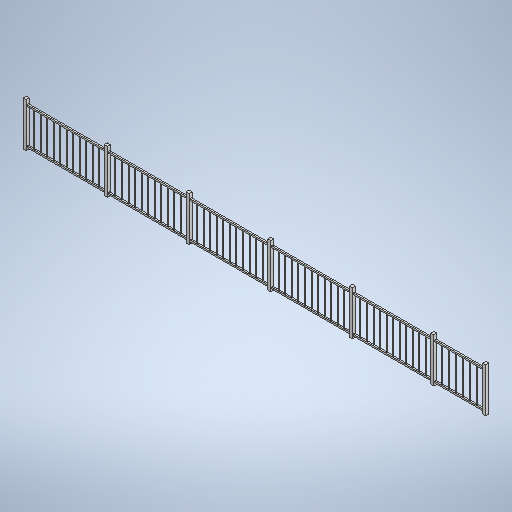
# Autodesk Inventor part: Railing Side B
Saved by Autodesk Inventor 2025 (Build 290162000, 162)
## iProperties
Created: 2024-07-15
Part Number: Railing Side B
Material: Generic
Document SubType Name: Modeling
Designer: track
Density: 1 g/cm^3
Appearance: Default
Author: track
Autodesk Inventor part; units mm, degrees
ref_plane "YZ Plane" through (0, 0, 0) normal (1, 0, 0) x (0, 1, 0)
ref_plane "XZ Plane" through (0, 0, 0) normal (0, 1, 0) x (-1, 0, 0)
ref_plane "XY Plane" through (0, 0, 0) normal (0, 0, 1) x (1, 0, 0)
sketch "Sketch1" plane through (0, 0, 0) normal (0, 1, 0) x (-1, 0, 0)
  line L0 (-38.1, -38.1) -> (38.1, -38.1)
  line L1 (38.1, -38.1) -> (38.1, 38.1)
  line L2 (38.1, 38.1) -> (-38.1, 38.1)
  line L3 (-38.1, 38.1) -> (-38.1, -38.1)
  line L4 (-38.1, -38.1) -> (38.1, 38.1) construction
  line L5 (38.1, -38.1) -> (-38.1, 38.1) construction
  point P0 (0, 0)
  dimension "d0" = 76.2
  dimension "d1" = 76.2
  constraints: 12 end point, 2 midpoint, 2 parallel, 1 horizontal, 1 perpendicular
  measures "d0" distance of L1.end L2.end
  measures "d1" distance of L0.end L1.end
extrude "Extrusion1" add sketch "Sketch1" along normal blind 1117.6
sketch "Sketch2" plane through (38.1, 0, 38.1) normal (1, 0, 0) x (0, 0, -1)
  line L0 (19.05, 95.25) -> (57.15, 95.25)
  line L1 (57.15, 95.25) -> (57.15, 57.15)
  line L2 (57.15, 57.15) -> (19.05, 57.15)
  line L3 (19.05, 57.15) -> (19.05, 95.25)
  line L4 (19.05, 95.25) -> (57.15, 57.15) construction
  line L5 (57.15, 95.25) -> (19.05, 57.15) construction
  line L6 (19.05, 996.95) -> (57.15, 996.95)
  line L7 (57.15, 996.95) -> (57.15, 958.85)
  line L8 (57.15, 958.85) -> (19.05, 958.85)
  line L9 (19.05, 958.85) -> (19.05, 996.95)
  line L10 (19.05, 996.95) -> (57.15, 958.85) construction
  line L11 (57.15, 996.95) -> (19.05, 958.85) construction
  line L12 (76.2, 329.1929) -> (76.2, 1461.8329)
  line L13 (76.2, 282.1305) -> (76.2, 1152.2607)
  line L14 (76.2, 0) -> (76.2, 1117.6) projected
  line L15 (0, 0) -> (76.2, 0) projected
  point P0 (38.1, 0)
  point P1 (-393.2293, 273.1932)
  point P2 (483.6892, 252.9929)
  point P3 (38.1, 76.2)
  point P4 (38.1, 977.9)
  dimension "d4" = 38.1
  dimension "d5" = 38.1
  dimension "d6" = 38.1
  dimension "d7" = 863.6
  dimension "d8" = 38.1
  dimension "d9" = 38.1
  dimension "d10" = 38.1
  dimension "d12" = 76.2
  constraints: 28 end point, 4 midpoint, 4 parallel, 2 horizontal, 2 perpendicular, 1 collinear, 1 point on line, 1 vertical
  measures "d4" distance of L0.end L1.end
  measures "d5" distance of L0.start L0.end
  measures "d6" distance from line of L12 point (38.1, 76.2)
  measures "d7" distance between parallel lines of L8 L0
  measures "d8" distance of L6.end L7.end
  measures "d9" distance of L6.start L6.end
  measures "d10" distance from line of L13 point (38.1, 977.9)
  measures "d12" distance from line of L15 point (38.1, 76.2)
extrude "Extrusion2" add sketch "Sketch2" along normal blind 1971.675
sketch "Sketch3" plane through (0, 0, 0) normal (0, 1, 0) x (-1, 0, 0)
  line L0 (0, 0) -> (-2047.875, 0)
  line L1 (-38.1, -19.05) -> (-2009.775, -19.05) projected
  line L2 (-2009.775, 38.1) -> (-2085.975, 38.1)
  line L3 (-2085.975, 38.1) -> (-2085.975, -38.1)
  line L4 (-2085.975, -38.1) -> (-2009.775, -38.1)
  line L5 (-2009.775, -38.1) -> (-2009.775, 38.1)
  line L6 (-2009.775, 38.1) -> (-2085.975, -38.1) construction
  line L7 (-2085.975, 38.1) -> (-2009.775, -38.1) construction
  line L8 (-2009.775, -19.05) -> (-2009.775, 19.05) projected
  dimension "d15" = 76.2
  dimension "d16" = 76.2
  constraints: 14 end point, 3 parallel, 2 midpoint, 1 collinear, 1 horizontal, 1 perpendicular
  measures "d15" distance of L3.end L4.end
  measures "d16" distance of L2.end L3.end
extrude "Extrusion3" add sketch "Sketch3" along normal blind 1117.6
sketch "Sketch4" plane through (2085.975, 0, 38.1) normal (1, 0, 0) x (0, 0, -1)
  line L0 (57.15, 996.95) -> (57.15, 958.85) projected
  line L1 (57.15, 958.85) -> (57.15, 996.95) projected
  line L2 (19.05, 996.95) -> (57.15, 996.95) projected
  line L3 (57.15, 996.95) -> (19.05, 996.95) projected
  line L4 (19.05, 958.85) -> (19.05, 996.95) projected
  line L5 (19.05, 996.95) -> (19.05, 958.85) projected
  line L6 (57.15, 958.85) -> (19.05, 958.85) projected
  line L7 (19.05, 958.85) -> (57.15, 958.85) projected
  line L8 (57.15, 57.15) -> (19.05, 57.15) projected
  line L9 (19.05, 57.15) -> (57.15, 57.15) projected
  line L10 (19.05, 57.15) -> (19.05, 95.25) projected
  line L11 (19.05, 95.25) -> (19.05, 57.15) projected
  line L12 (19.05, 95.25) -> (57.15, 95.25) projected
  line L13 (57.15, 95.25) -> (19.05, 95.25) projected
  line L14 (57.15, 95.25) -> (57.15, 57.15) projected
  line L15 (57.15, 57.15) -> (57.15, 95.25) projected
  line L16 (19.05, 95.25) -> (57.15, 95.25)
  line L17 (57.15, 95.25) -> (57.15, 57.15)
  line L18 (57.15, 57.15) -> (19.05, 57.15)
  line L19 (19.05, 57.15) -> (19.05, 95.25)
  line L20 (19.05, 996.95) -> (57.15, 996.95)
  line L21 (57.15, 996.95) -> (57.15, 958.85)
  line L22 (57.15, 958.85) -> (19.05, 958.85)
  line L23 (19.05, 958.85) -> (19.05, 996.95)
  point P0 (38.1, 0)
  point P1 (19.05, 958.85)
  point P2 (57.15, 958.85)
  point P3 (57.15, 996.95)
  point P4 (19.05, 996.95)
  point P5 (57.15, 57.15)
  point P6 (57.15, 95.25)
  point P7 (19.05, 95.25)
  point P8 (19.05, 57.15)
  constraints: 16 end point, 4 parallel, 2 horizontal, 2 perpendicular
extrude "Extrusion4" add sketch "Sketch4" along normal blind 1985.9625
sketch "Sketch5" plane through (0, 0, 0) normal (0, 1, 0) x (-1, 0, 0)
  line L0 (-4071.9375, -19.05) -> (-4071.9375, 19.05) projected
  line L1 (-4071.9375, 0) -> (-4110.0375, 0)
  line L2 (-4148.1375, -38.1) -> (-4071.9375, -38.1)
  line L3 (-4071.9375, -38.1) -> (-4071.9375, 38.1)
  line L4 (-4071.9375, 38.1) -> (-4148.1375, 38.1)
  line L5 (-4148.1375, 38.1) -> (-4148.1375, -38.1)
  line L6 (-4148.1375, -38.1) -> (-4071.9375, 38.1) construction
  line L7 (-4071.9375, -38.1) -> (-4148.1375, 38.1) construction
  line L8 (-4071.9375, -19.05) -> (-4071.9375, 19.05) projected
  point P0 (0, 0)
  dimension "d21" = 76.2
  dimension "d22" = 76.2
  constraints: 14 end point, 3 midpoint, 2 horizontal, 2 parallel, 1 collinear, 1 perpendicular
  measures "d21" distance of L2.start L2.end
  measures "d22" distance of L4.end L2.start
extrude "Extrusion5" add sketch "Sketch5" along normal blind 1117.6
sketch "Sketch6" plane through (4148.1375, 0, 38.1) normal (1, 0, 0) x (0, 0, -1)
  line L0 (19.05, 95.25) -> (57.15, 95.25) projected
  line L1 (57.15, 95.25) -> (19.05, 95.25) projected
  line L2 (19.05, 57.15) -> (19.05, 95.25) projected
  line L3 (19.05, 95.25) -> (19.05, 57.15) projected
  line L4 (57.15, 95.25) -> (57.15, 57.15) projected
  line L5 (57.15, 57.15) -> (57.15, 95.25) projected
  line L6 (57.15, 57.15) -> (19.05, 57.15) projected
  line L7 (19.05, 57.15) -> (57.15, 57.15) projected
  line L8 (57.15, 996.95) -> (57.15, 958.85) projected
  line L9 (57.15, 958.85) -> (57.15, 996.95) projected
  line L10 (57.15, 958.85) -> (19.05, 958.85) projected
  line L11 (19.05, 958.85) -> (57.15, 958.85) projected
  line L12 (19.05, 996.95) -> (57.15, 996.95) projected
  line L13 (57.15, 996.95) -> (19.05, 996.95) projected
  line L14 (19.05, 958.85) -> (19.05, 996.95) projected
  line L15 (19.05, 996.95) -> (19.05, 958.85) projected
  point P0 (38.1, 0)
extrude "Extrusion6" add sketch "Sketch6" along normal blind 1984.375
sketch "Sketch7" plane through (0, 0, 0) normal (0, 1, 0) x (-1, 0, 0)
  line L0 (-6132.5125, 19.05) -> (-6132.5125, -19.05) projected
  line L1 (-6132.5125, 0) -> (-6170.6125, 0)
  line L2 (-6132.5125, 38.1) -> (-6208.7125, 38.1)
  line L3 (-6208.7125, 38.1) -> (-6208.7125, -38.1)
  line L4 (-6208.7125, -38.1) -> (-6132.5125, -38.1)
  line L5 (-6132.5125, -38.1) -> (-6132.5125, 38.1)
  line L6 (-6132.5125, 38.1) -> (-6208.7125, -38.1) construction
  line L7 (-6208.7125, 38.1) -> (-6132.5125, -38.1) construction
  line L8 (-6132.5125, -19.05) -> (-6132.5125, 19.05) projected
  point P0 (0, 0)
  dimension "d27" = 76.2
  dimension "d28" = 76.2
  constraints: 14 end point, 3 midpoint, 2 horizontal, 2 parallel, 1 collinear, 1 perpendicular
  measures "d27" distance of L4.end L2.start
  measures "d28" distance of L3.end L4.end
extrude "Extrusion7" add sketch "Sketch7" along normal blind 1117.6
sketch "Sketch8" plane through (6208.7125, 0, 38.1) normal (1, 0, 0) x (0, 0, -1)
  line L0 (19.05, 958.85) -> (19.05, 996.95) projected
  line L1 (19.05, 996.95) -> (19.05, 958.85) projected
  line L2 (19.05, 996.95) -> (57.15, 996.95) projected
  line L3 (57.15, 996.95) -> (19.05, 996.95) projected
  line L4 (57.15, 996.95) -> (57.15, 958.85) projected
  line L5 (57.15, 958.85) -> (57.15, 996.95) projected
  line L6 (57.15, 958.85) -> (19.05, 958.85) projected
  line L7 (19.05, 958.85) -> (57.15, 958.85) projected
  line L8 (57.15, 95.25) -> (57.15, 57.15) projected
  line L9 (57.15, 57.15) -> (57.15, 95.25) projected
  line L10 (57.15, 57.15) -> (19.05, 57.15) projected
  line L11 (19.05, 57.15) -> (57.15, 57.15) projected
  line L12 (19.05, 95.25) -> (57.15, 95.25) projected
  line L13 (57.15, 95.25) -> (19.05, 95.25) projected
  line L14 (19.05, 57.15) -> (19.05, 95.25) projected
  line L15 (19.05, 95.25) -> (19.05, 57.15) projected
  point P0 (38.1, 0)
extrude "Extrusion8" add sketch "Sketch8" along normal blind 1984.375
sketch "Sketch9" plane through (0, 0, 0) normal (0, 1, 0) x (-1, 0, 0)
  line L0 (-8193.0875, 19.05) -> (-8193.0875, -19.05) projected
  line L1 (-8193.0875, 0) -> (-8231.1875, 0)
  line L2 (-8193.0875, 38.1) -> (-8269.2875, 38.1)
  line L3 (-8269.2875, 38.1) -> (-8269.2875, -38.1)
  line L4 (-8269.2875, -38.1) -> (-8193.0875, -38.1)
  line L5 (-8193.0875, -38.1) -> (-8193.0875, 38.1)
  line L6 (-8193.0875, 38.1) -> (-8269.2875, -38.1) construction
  line L7 (-8269.2875, 38.1) -> (-8193.0875, -38.1) construction
  line L8 (-8193.0875, -19.05) -> (-8193.0875, 19.05) projected
  point P0 (0, 0)
  dimension "d33" = 76.2
  dimension "d34" = 76.2
  constraints: 14 end point, 3 midpoint, 2 horizontal, 2 parallel, 1 collinear, 1 perpendicular
  measures "d33" distance of L3.end L4.end
  measures "d34" distance of L4.end L2.start
extrude "Extrusion9" add sketch "Sketch9" along normal blind 1117.6
sketch "Sketch10" plane through (8269.2875, 0, 38.1) normal (1, 0, 0) x (0, 0, -1)
  line L0 (19.05, 57.15) -> (19.05, 95.25) projected
  line L1 (19.05, 95.25) -> (19.05, 57.15) projected
  line L2 (19.05, 95.25) -> (57.15, 95.25) projected
  line L3 (57.15, 95.25) -> (19.05, 95.25) projected
  line L4 (57.15, 95.25) -> (57.15, 57.15) projected
  line L5 (57.15, 57.15) -> (57.15, 95.25) projected
  line L6 (57.15, 57.15) -> (19.05, 57.15) projected
  line L7 (19.05, 57.15) -> (57.15, 57.15) projected
  line L8 (57.15, 958.85) -> (19.05, 958.85) projected
  line L9 (19.05, 958.85) -> (57.15, 958.85) projected
  line L10 (57.15, 996.95) -> (57.15, 958.85) projected
  line L11 (57.15, 958.85) -> (57.15, 996.95) projected
  line L12 (19.05, 996.95) -> (57.15, 996.95) projected
  line L13 (57.15, 996.95) -> (19.05, 996.95) projected
  line L14 (19.05, 958.85) -> (19.05, 996.95) projected
  line L15 (19.05, 996.95) -> (19.05, 958.85) projected
  point P0 (38.1, 0)
extrude "Extrusion10" add sketch "Sketch10" along normal blind 1981.2
sketch "Sketch11" plane through (0, 0, 0) normal (0, 1, 0) x (-1, 0, 0)
  line L0 (-10250.4875, 19.05) -> (-10250.4875, -19.05) projected
  line L1 (-10250.4875, 0) -> (-10288.5875, 0)
  line L2 (-10326.6875, 38.1) -> (-10250.4875, 38.1)
  line L3 (-10250.4875, 38.1) -> (-10250.4875, -38.1)
  line L4 (-10250.4875, -38.1) -> (-10326.6875, -38.1)
  line L5 (-10326.6875, -38.1) -> (-10326.6875, 38.1)
  line L6 (-10326.6875, 38.1) -> (-10250.4875, -38.1) construction
  line L7 (-10250.4875, 38.1) -> (-10326.6875, -38.1) construction
  line L8 (-10250.4875, -19.05) -> (-10250.4875, 19.05) projected
  point P0 (0, 0)
  dimension "d39" = 76.2
  dimension "d40" = 76.2
  constraints: 14 end point, 3 midpoint, 2 horizontal, 2 parallel, 1 collinear, 1 perpendicular
  measures "d39" distance of L4.end L2.start
  measures "d40" distance of L3.end L4.end
extrude "Extrusion11" add sketch "Sketch11" along normal blind 1117.6
sketch "Sketch12" plane through (10326.6875, 0, 38.1) normal (1, 0, 0) x (0, 0, -1)
  line L0 (19.05, 57.15) -> (19.05, 95.25) projected
  line L1 (19.05, 95.25) -> (19.05, 57.15) projected
  line L2 (19.05, 95.25) -> (57.15, 95.25) projected
  line L3 (57.15, 95.25) -> (19.05, 95.25) projected
  line L4 (57.15, 95.25) -> (57.15, 57.15) projected
  line L5 (57.15, 57.15) -> (57.15, 95.25) projected
  line L6 (57.15, 57.15) -> (19.05, 57.15) projected
  line L7 (19.05, 57.15) -> (57.15, 57.15) projected
  line L8 (57.15, 958.85) -> (19.05, 958.85) projected
  line L9 (19.05, 958.85) -> (57.15, 958.85) projected
  line L10 (57.15, 996.95) -> (57.15, 958.85) projected
  line L11 (57.15, 958.85) -> (57.15, 996.95) projected
  line L12 (19.05, 996.95) -> (57.15, 996.95) projected
  line L13 (57.15, 996.95) -> (19.05, 996.95) projected
  line L14 (19.05, 958.85) -> (19.05, 996.95) projected
  line L15 (19.05, 996.95) -> (19.05, 958.85) projected
  point P0 (38.1, 0)
  point P1 (76.2, 0)
  point P2 (19.05, 57.15)
  point P3 (57.15, 57.15)
  point P4 (57.15, 95.25)
  point P5 (19.05, 95.25)
  point P6 (19.05, 996.95)
  point P7 (19.05, 958.85)
  point P8 (57.15, 958.85)
  point P9 (57.15, 996.95)
extrude "Extrusion12" add sketch "Sketch12" along normal blind 1231.9
sketch "Sketch13" plane through (0, 0, 0) normal (0, 1, 0) x (-1, 0, 0)
  line L0 (-11558.5875, 19.05) -> (-11558.5875, -19.05) projected
  line L1 (-11558.5875, 0) -> (-11596.6875, 0)
  line L2 (-11558.5875, 38.1) -> (-11634.7875, 38.1)
  line L3 (-11634.7875, 38.1) -> (-11634.7875, -38.1)
  line L4 (-11634.7875, -38.1) -> (-11558.5875, -38.1)
  line L5 (-11558.5875, -38.1) -> (-11558.5875, 38.1)
  line L6 (-11558.5875, 38.1) -> (-11634.7875, -38.1) construction
  line L7 (-11634.7875, 38.1) -> (-11558.5875, -38.1) construction
  line L8 (-11558.5875, -19.05) -> (-11558.5875, 19.05) projected
  point P0 (0, 0)
  dimension "d45" = 76.2
  dimension "d46" = 76.2
  constraints: 14 end point, 3 midpoint, 2 horizontal, 2 parallel, 1 collinear, 1 perpendicular
  measures "d45" distance of L3.end L4.end
  measures "d46" distance of L2.end L3.end
extrude "Extrusion13" add sketch "Sketch13" along normal blind 1117.6
sketch "Sketch14" plane through (38.1, 95.25, 19.05) normal (0, 1, 0) x (1, 0, 0)
  line L0 (0, 0) -> (0, 38.1) projected
  line L1 (0, 19.05) -> (11596.6875, 19.05) construction
  line L2 (11596.6875, -19.05) -> (11596.6875, 57.15) projected
  line L3 (157.9562, 12.7) -> (170.6562, 12.7)
  line L4 (170.6562, 12.7) -> (170.6562, 25.4)
  line L5 (170.6562, 25.4) -> (157.9562, 25.4)
  line L6 (157.9562, 25.4) -> (157.9562, 12.7)
  line L7 (157.9562, 12.7) -> (170.6562, 25.4) construction
  line L8 (170.6562, 12.7) -> (157.9562, 25.4) construction
  line L9 (322.2625, 12.7) -> (334.9625, 12.7)
  line L10 (334.9625, 12.7) -> (334.9625, 25.4)
  line L11 (334.9625, 25.4) -> (322.2625, 25.4)
  line L12 (322.2625, 25.4) -> (322.2625, 12.7)
  line L13 (486.5687, 12.7) -> (499.2687, 12.7)
  line L14 (499.2687, 12.7) -> (499.2687, 25.4)
  line L15 (499.2687, 25.4) -> (486.5687, 25.4)
  line L16 (486.5687, 25.4) -> (486.5687, 12.7)
  line L17 (650.875, 12.7) -> (663.575, 12.7)
  line L18 (663.575, 12.7) -> (663.575, 25.4)
  line L19 (663.575, 25.4) -> (650.875, 25.4)
  line L20 (650.875, 25.4) -> (650.875, 12.7)
  line L21 (815.1812, 12.7) -> (827.8812, 12.7)
  line L22 (827.8812, 12.7) -> (827.8812, 25.4)
  line L23 (827.8812, 25.4) -> (815.1812, 25.4)
  line L24 (815.1812, 25.4) -> (815.1812, 12.7)
  line L25 (979.4875, 12.7) -> (992.1875, 12.7)
  line L26 (992.1875, 12.7) -> (992.1875, 25.4)
  line L27 (992.1875, 25.4) -> (979.4875, 25.4)
  line L28 (979.4875, 25.4) -> (979.4875, 12.7)
  line L29 (1143.7937, 12.7) -> (1156.4937, 12.7)
  line L30 (1156.4937, 12.7) -> (1156.4937, 25.4)
  line L31 (1156.4937, 25.4) -> (1143.7937, 25.4)
  line L32 (1143.7937, 25.4) -> (1143.7937, 12.7)
  line L33 (1308.1, 12.7) -> (1320.8, 12.7)
  line L34 (1320.8, 12.7) -> (1320.8, 25.4)
  line L35 (1320.8, 25.4) -> (1308.1, 25.4)
  line L36 (1308.1, 25.4) -> (1308.1, 12.7)
  line L37 (1472.4062, 12.7) -> (1485.1062, 12.7)
  line L38 (1485.1062, 12.7) -> (1485.1062, 25.4)
  line L39 (1485.1062, 25.4) -> (1472.4062, 25.4)
  line L40 (1472.4062, 25.4) -> (1472.4062, 12.7)
  line L41 (1636.7125, 12.7) -> (1649.4125, 12.7)
  line L42 (1649.4125, 12.7) -> (1649.4125, 25.4)
  line L43 (1649.4125, 25.4) -> (1636.7125, 25.4)
  line L44 (1636.7125, 25.4) -> (1636.7125, 12.7)
  line L45 (1801.0187, 12.7) -> (1813.7187, 12.7)
  line L46 (1813.7187, 12.7) -> (1813.7187, 25.4)
  line L47 (1813.7187, 25.4) -> (1801.0187, 25.4)
  line L48 (1801.0187, 25.4) -> (1801.0187, 12.7)
  line L49 (2207.0219, 12.7) -> (2219.7219, 12.7)
  line L50 (2219.7219, 12.7) -> (2219.7219, 25.4)
  line L51 (2219.7219, 25.4) -> (2207.0219, 25.4)
  line L52 (2207.0219, 25.4) -> (2207.0219, 12.7)
  line L53 (2207.0219, 12.7) -> (2219.7219, 25.4) construction
  line L54 (2219.7219, 12.7) -> (2207.0219, 25.4) construction
  line L55 (2047.875, 0) -> (2047.875, 38.1) projected
  line L56 (2385.2187, 25.4) -> (2372.5187, 25.4)
  line L57 (2372.5187, 25.4) -> (2372.5187, 12.7)
  line L58 (2385.2187, 12.7) -> (2385.2187, 25.4)
  line L59 (2372.5187, 12.7) -> (2385.2187, 12.7)
  line L60 (2550.7156, 25.4) -> (2538.0156, 25.4)
  line L61 (2538.0156, 25.4) -> (2538.0156, 12.7)
  line L62 (2550.7156, 12.7) -> (2550.7156, 25.4)
  line L63 (2538.0156, 12.7) -> (2550.7156, 12.7)
  line L64 (2716.2125, 25.4) -> (2703.5125, 25.4)
  line L65 (2703.5125, 25.4) -> (2703.5125, 12.7)
  line L66 (2716.2125, 12.7) -> (2716.2125, 25.4)
  line L67 (2703.5125, 12.7) -> (2716.2125, 12.7)
  line L68 (2881.7094, 25.4) -> (2869.0094, 25.4)
  line L69 (2869.0094, 25.4) -> (2869.0094, 12.7)
  line L70 (2881.7094, 12.7) -> (2881.7094, 25.4)
  line L71 (2869.0094, 12.7) -> (2881.7094, 12.7)
  line L72 (3047.2062, 25.4) -> (3034.5062, 25.4)
  line L73 (3034.5062, 25.4) -> (3034.5062, 12.7)
  line L74 (3047.2062, 12.7) -> (3047.2062, 25.4)
  line L75 (3034.5062, 12.7) -> (3047.2062, 12.7)
  line L76 (3212.7031, 25.4) -> (3200.0031, 25.4)
  line L77 (3200.0031, 25.4) -> (3200.0031, 12.7)
  line L78 (3212.7031, 12.7) -> (3212.7031, 25.4)
  line L79 (3200.0031, 12.7) -> (3212.7031, 12.7)
  line L80 (3378.2, 25.4) -> (3365.5, 25.4)
  line L81 (3365.5, 25.4) -> (3365.5, 12.7)
  line L82 (3378.2, 12.7) -> (3378.2, 25.4)
  line L83 (3365.5, 12.7) -> (3378.2, 12.7)
  line L84 (3543.6969, 25.4) -> (3530.9969, 25.4)
  line L85 (3530.9969, 25.4) -> (3530.9969, 12.7)
  line L86 (3543.6969, 12.7) -> (3543.6969, 25.4)
  line L87 (3530.9969, 12.7) -> (3543.6969, 12.7)
  line L88 (3709.1937, 25.4) -> (3696.4937, 25.4)
  line L89 (3696.4937, 25.4) -> (3696.4937, 12.7)
  line L90 (3709.1937, 12.7) -> (3709.1937, 25.4)
  line L91 (3696.4937, 12.7) -> (3709.1937, 12.7)
  line L92 (3874.6906, 25.4) -> (3861.9906, 25.4)
  line L93 (3861.9906, 25.4) -> (3861.9906, 12.7)
  line L94 (3874.6906, 12.7) -> (3874.6906, 25.4)
  line L95 (3861.9906, 12.7) -> (3874.6906, 12.7)
  line L96 (4269.0521, 12.7) -> (4281.7521, 12.7)
  line L97 (4281.7521, 12.7) -> (4281.7521, 25.4)
  line L98 (4281.7521, 25.4) -> (4269.0521, 25.4)
  line L99 (4269.0521, 25.4) -> (4269.0521, 12.7)
  line L100 (4269.0521, 12.7) -> (4281.7521, 25.4) construction
  line L101 (4281.7521, 12.7) -> (4269.0521, 25.4) construction
  line L102 (4110.0375, 0) -> (4110.0375, 38.1) projected
  line L103 (4447.1167, 12.7) -> (4447.1167, 25.4)
  line L104 (4447.1167, 25.4) -> (4434.4167, 25.4)
  line L105 (4434.4167, 25.4) -> (4434.4167, 12.7)
  line L106 (4434.4167, 12.7) -> (4447.1167, 12.7)
  line L107 (4612.4812, 12.7) -> (4612.4812, 25.4)
  line L108 (4612.4812, 25.4) -> (4599.7812, 25.4)
  line L109 (4599.7812, 25.4) -> (4599.7812, 12.7)
  line L110 (4599.7812, 12.7) -> (4612.4812, 12.7)
  line L111 (4777.8458, 12.7) -> (4777.8458, 25.4)
  line L112 (4777.8458, 25.4) -> (4765.1458, 25.4)
  line L113 (4765.1458, 25.4) -> (4765.1458, 12.7)
  line L114 (4765.1458, 12.7) -> (4777.8458, 12.7)
  line L115 (4943.2104, 12.7) -> (4943.2104, 25.4)
  line L116 (4943.2104, 25.4) -> (4930.5104, 25.4)
  line L117 (4930.5104, 25.4) -> (4930.5104, 12.7)
  line L118 (4930.5104, 12.7) -> (4943.2104, 12.7)
  line L119 (5108.575, 12.7) -> (5108.575, 25.4)
  line L120 (5108.575, 25.4) -> (5095.875, 25.4)
  line L121 (5095.875, 25.4) -> (5095.875, 12.7)
  line L122 (5095.875, 12.7) -> (5108.575, 12.7)
  line L123 (5273.9396, 12.7) -> (5273.9396, 25.4)
  line L124 (5273.9396, 25.4) -> (5261.2396, 25.4)
  line L125 (5261.2396, 25.4) -> (5261.2396, 12.7)
  line L126 (5261.2396, 12.7) -> (5273.9396, 12.7)
  line L127 (5439.3042, 12.7) -> (5439.3042, 25.4)
  line L128 (5439.3042, 25.4) -> (5426.6042, 25.4)
  line L129 (5426.6042, 25.4) -> (5426.6042, 12.7)
  line L130 (5426.6042, 12.7) -> (5439.3042, 12.7)
  line L131 (5604.6687, 12.7) -> (5604.6687, 25.4)
  line L132 (5604.6687, 25.4) -> (5591.9688, 25.4)
  line L133 (5591.9688, 25.4) -> (5591.9688, 12.7)
  line L134 (5591.9688, 12.7) -> (5604.6687, 12.7)
  line L135 (5770.0333, 12.7) -> (5770.0333, 25.4)
  line L136 (5770.0333, 25.4) -> (5757.3333, 25.4)
  line L137 (5757.3333, 25.4) -> (5757.3333, 12.7)
  line L138 (5757.3333, 12.7) -> (5770.0333, 12.7)
  line L139 (5935.3979, 12.7) -> (5935.3979, 25.4)
  line L140 (5935.3979, 25.4) -> (5922.6979, 25.4)
  line L141 (5922.6979, 25.4) -> (5922.6979, 12.7)
  line L142 (5922.6979, 12.7) -> (5935.3979, 12.7)
  line L143 (6329.6271, 12.7) -> (6342.3271, 12.7)
  line L144 (6342.3271, 12.7) -> (6342.3271, 25.4)
  line L145 (6342.3271, 25.4) -> (6329.6271, 25.4)
  line L146 (6329.6271, 25.4) -> (6329.6271, 12.7)
  line L147 (6329.6271, 12.7) -> (6342.3271, 25.4) construction
  line L148 (6342.3271, 12.7) -> (6329.6271, 25.4) construction
  line L149 (6170.6125, 0) -> (6170.6125, 38.1) projected
  line L150 (6507.6917, 25.4) -> (6494.9917, 25.4)
  line L151 (6507.6917, 12.7) -> (6507.6917, 25.4)
  line L152 (6494.9917, 25.4) -> (6494.9917, 12.7)
  line L153 (6494.9917, 12.7) -> (6507.6917, 12.7)
  line L154 (6673.0563, 25.4) -> (6660.3563, 25.4)
  line L155 (6673.0563, 12.7) -> (6673.0563, 25.4)
  line L156 (6660.3563, 25.4) -> (6660.3563, 12.7)
  line L157 (6660.3563, 12.7) -> (6673.0563, 12.7)
  line L158 (6838.4208, 25.4) -> (6825.7208, 25.4)
  line L159 (6838.4208, 12.7) -> (6838.4208, 25.4)
  line L160 (6825.7208, 25.4) -> (6825.7208, 12.7)
  line L161 (6825.7208, 12.7) -> (6838.4208, 12.7)
  line L162 (7003.7854, 25.4) -> (6991.0854, 25.4)
  line L163 (7003.7854, 12.7) -> (7003.7854, 25.4)
  line L164 (6991.0854, 25.4) -> (6991.0854, 12.7)
  line L165 (6991.0854, 12.7) -> (7003.7854, 12.7)
  line L166 (7169.15, 25.4) -> (7156.45, 25.4)
  line L167 (7169.15, 12.7) -> (7169.15, 25.4)
  line L168 (7156.45, 25.4) -> (7156.45, 12.7)
  line L169 (7156.45, 12.7) -> (7169.15, 12.7)
  line L170 (7334.5146, 25.4) -> (7321.8146, 25.4)
  line L171 (7334.5146, 12.7) -> (7334.5146, 25.4)
  line L172 (7321.8146, 25.4) -> (7321.8146, 12.7)
  line L173 (7321.8146, 12.7) -> (7334.5146, 12.7)
  line L174 (7499.8792, 25.4) -> (7487.1792, 25.4)
  line L175 (7499.8792, 12.7) -> (7499.8792, 25.4)
  line L176 (7487.1792, 25.4) -> (7487.1792, 12.7)
  line L177 (7487.1792, 12.7) -> (7499.8792, 12.7)
  line L178 (7665.2438, 25.4) -> (7652.5438, 25.4)
  line L179 (7665.2438, 12.7) -> (7665.2438, 25.4)
  line L180 (7652.5438, 25.4) -> (7652.5438, 12.7)
  line L181 (7652.5438, 12.7) -> (7665.2438, 12.7)
  line L182 (7830.6083, 25.4) -> (7817.9083, 25.4)
  line L183 (7830.6083, 12.7) -> (7830.6083, 25.4)
  line L184 (7817.9083, 25.4) -> (7817.9083, 12.7)
  line L185 (7817.9083, 12.7) -> (7830.6083, 12.7)
  line L186 (7995.9729, 25.4) -> (7983.2729, 25.4)
  line L187 (7995.9729, 12.7) -> (7995.9729, 25.4)
  line L188 (7983.2729, 25.4) -> (7983.2729, 12.7)
  line L189 (7983.2729, 12.7) -> (7995.9729, 12.7)
  line L190 (8389.9375, 12.7) -> (8402.6375, 12.7)
  line L191 (8402.6375, 12.7) -> (8402.6375, 25.4)
  line L192 (8402.6375, 25.4) -> (8389.9375, 25.4)
  line L193 (8389.9375, 25.4) -> (8389.9375, 12.7)
  line L194 (8389.9375, 12.7) -> (8402.6375, 25.4) construction
  line L195 (8402.6375, 12.7) -> (8389.9375, 25.4) construction
  line L196 (8231.1875, 0) -> (8231.1875, 38.1) projected
  line L197 (8567.7375, 12.7) -> (8567.7375, 25.4)
  line L198 (8567.7375, 25.4) -> (8555.0375, 25.4)
  line L199 (8555.0375, 25.4) -> (8555.0375, 12.7)
  line L200 (8555.0375, 12.7) -> (8567.7375, 12.7)
  line L201 (8732.8375, 12.7) -> (8732.8375, 25.4)
  line L202 (8732.8375, 25.4) -> (8720.1375, 25.4)
  line L203 (8720.1375, 25.4) -> (8720.1375, 12.7)
  line L204 (8720.1375, 12.7) -> (8732.8375, 12.7)
  line L205 (8897.9375, 12.7) -> (8897.9375, 25.4)
  line L206 (8897.9375, 25.4) -> (8885.2375, 25.4)
  line L207 (8885.2375, 25.4) -> (8885.2375, 12.7)
  line L208 (8885.2375, 12.7) -> (8897.9375, 12.7)
  line L209 (9063.0375, 12.7) -> (9063.0375, 25.4)
  line L210 (9063.0375, 25.4) -> (9050.3375, 25.4)
  line L211 (9050.3375, 25.4) -> (9050.3375, 12.7)
  line L212 (9050.3375, 12.7) -> (9063.0375, 12.7)
  line L213 (9228.1375, 12.7) -> (9228.1375, 25.4)
  line L214 (9228.1375, 25.4) -> (9215.4375, 25.4)
  line L215 (9215.4375, 25.4) -> (9215.4375, 12.7)
  line L216 (9215.4375, 12.7) -> (9228.1375, 12.7)
  line L217 (9393.2375, 12.7) -> (9393.2375, 25.4)
  line L218 (9393.2375, 25.4) -> (9380.5375, 25.4)
  line L219 (9380.5375, 25.4) -> (9380.5375, 12.7)
  line L220 (9380.5375, 12.7) -> (9393.2375, 12.7)
  line L221 (9558.3375, 12.7) -> (9558.3375, 25.4)
  line L222 (9558.3375, 25.4) -> (9545.6375, 25.4)
  line L223 (9545.6375, 25.4) -> (9545.6375, 12.7)
  line L224 (9545.6375, 12.7) -> (9558.3375, 12.7)
  line L225 (9723.4375, 12.7) -> (9723.4375, 25.4)
  line L226 (9723.4375, 25.4) -> (9710.7375, 25.4)
  line L227 (9710.7375, 25.4) -> (9710.7375, 12.7)
  line L228 (9710.7375, 12.7) -> (9723.4375, 12.7)
  line L229 (9888.5375, 12.7) -> (9888.5375, 25.4)
  line L230 (9888.5375, 25.4) -> (9875.8375, 25.4)
  line L231 (9875.8375, 25.4) -> (9875.8375, 12.7)
  line L232 (9875.8375, 12.7) -> (9888.5375, 12.7)
  line L233 (10053.6375, 12.7) -> (10053.6375, 25.4)
  line L234 (10053.6375, 25.4) -> (10040.9375, 25.4)
  line L235 (10040.9375, 25.4) -> (10040.9375, 12.7)
  line L236 (10040.9375, 12.7) -> (10053.6375, 12.7)
  line L237 (10458.2232, 12.7) -> (10470.9232, 12.7)
  line L238 (10470.9232, 12.7) -> (10470.9232, 25.4)
  line L239 (10470.9232, 25.4) -> (10458.2232, 25.4)
  line L240 (10458.2232, 25.4) -> (10458.2232, 12.7)
  line L241 (10458.2232, 12.7) -> (10470.9232, 25.4) construction
  line L242 (10470.9232, 12.7) -> (10458.2232, 25.4) construction
  line L243 (10288.5875, 0) -> (10288.5875, 38.1) projected
  line L244 (10646.9089, 12.7) -> (10646.9089, 25.4)
  line L245 (10646.9089, 25.4) -> (10634.2089, 25.4)
  line L246 (10634.2089, 25.4) -> (10634.2089, 12.7)
  line L247 (10634.2089, 12.7) -> (10646.9089, 12.7)
  line L248 (10822.8946, 12.7) -> (10822.8946, 25.4)
  line L249 (10822.8946, 25.4) -> (10810.1946, 25.4)
  line L250 (10810.1946, 25.4) -> (10810.1946, 12.7)
  line L251 (10810.1946, 12.7) -> (10822.8946, 12.7)
  line L252 (10998.8804, 12.7) -> (10998.8804, 25.4)
  line L253 (10998.8804, 25.4) -> (10986.1804, 25.4)
  line L254 (10986.1804, 25.4) -> (10986.1804, 12.7)
  line L255 (10986.1804, 12.7) -> (10998.8804, 12.7)
  line L256 (11174.8661, 12.7) -> (11174.8661, 25.4)
  line L257 (11174.8661, 25.4) -> (11162.1661, 25.4)
  line L258 (11162.1661, 25.4) -> (11162.1661, 12.7)
  line L259 (11162.1661, 12.7) -> (11174.8661, 12.7)
  line L260 (11350.8518, 12.7) -> (11350.8518, 25.4)
  line L261 (11350.8518, 25.4) -> (11338.1518, 25.4)
  line L262 (11338.1518, 25.4) -> (11338.1518, 12.7)
  line L263 (11338.1518, 12.7) -> (11350.8518, 12.7)
  point P0 (-38.1, 19.05)
  point P1 (164.3062, 19.05)
  point P2 (2213.3719, 19.05)
  point P3 (4275.4021, 19.05)
  point P4 (6335.9771, 19.05)
  point P5 (8396.2875, 19.05)
  point P6 (10464.5732, 19.05)
  dimension "d49" = 12.7
  dimension "d50" = 12.7
  dimension "d51" = 164.3063
  dimension "d54" = 164.3063
  dimension "d59" = 12.7
  dimension "d60" = 12.7
  dimension "d61" = 165.4969
  dimension "d64" = 165.4969
  dimension "d69" = 12.7
  dimension "d70" = 12.7
  dimension "d71" = 165.3646
  dimension "d74" = 165.3646
  dimension "d79" = 12.7
  dimension "d80" = 12.7
  dimension "d81" = 165.3646
  dimension "d84" = 165.3646
  dimension "d89" = 12.7
  dimension "d90" = 12.7
  dimension "d91" = 165.1
  dimension "d94" = 165.1
  dimension "d99" = 12.7
  dimension "d100" = 12.7
  dimension "d101" = 175.9857
  dimension "d104" = 175.9857
  constraints: 514 end point, 14 midpoint, 12 horizontal, 12 parallel, 6 perpendicular, 6 point on line, 440 other
  measures "d49" distance of L4.end L5.end
  measures "d50" distance of L3.end L4.end
  measures "d51" distance from line of L0 point (164.306, 19.05)
  measures "d54" distance of L3.start L9.start
  measures "d59" distance of L50.end L51.end
  measures "d60" distance of L49.end L50.end
  measures "d61" distance from line of L55 point (2213.372, 19.05)
  measures "d64" distance of L50.end L56.start
  measures "d69" distance of L97.end L98.end
  measures "d70" distance of L96.end L97.end
  measures "d71" distance from line of L102 point (4275.402, 19.05)
  measures "d74" distance of L96.end L103.start
  measures "d79" distance of L144.end L145.end
  measures "d80" distance of L143.end L144.end
  measures "d81" distance from line of L149 point (6335.977, 19.05)
  measures "d84" distance of L144.end L150.start
  measures "d89" distance of L191.end L192.end
  measures "d90" distance of L190.end L191.end
  measures "d91" distance from line of L196 point (8396.288, 19.05)
  measures "d94" distance of L190.end L197.start
  measures "d99" distance of L238.end L239.end
  measures "d100" distance of L237.end L238.end
  measures "d101" distance from line of L243 point (10464.573, 19.05)
  measures "d104" distance of L237.end L244.start
extrude "Extrusion14" add sketch "Sketch14" along normal up to surface (863.6 mm away)
body "Solid1"
